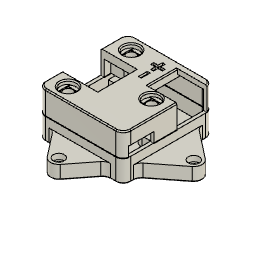
USB Adapter Mount (Autodesk Fusion 360 design; units mm, degrees)
Autodesk Fusion 360 part; units mm, degrees
note: some values were not read from the file. Chosen so that the rebuilt part matches the saved one: which face or edge a step refers to; which pieces of a blend or face edit are solid.
(part 1 of 2)
sketch "Sketch1" plane through (0, 0, 0) normal (0, 0, 1) x (1, 0, 0) in component "PCB"
  line L0 (0, 0) -> (27.432, 0)
  line L1 (27.432, 0) -> (27.432, 29.845)
  line L2 (27.432, 29.845) -> (0, 29.845)
  line L3 (0, 29.845) -> (0, 0)
  circle A0 centre (4.5, 3.5473) radius 1.6
  circle A1 centre (4.5, 26.5343) radius 1.6
  circle A2 centre (23.596, 14.865) radius 1.6
  line L4 (4.5, 26.5343) -> (4.5, 3.5473) construction
  dimension "d1" = 29.845
  dimension "d2" = 27.432
  dimension "d3" = 3.2
  dimension "d4" = 3.836
  dimension "d5" = 14.865
  dimension "d6" = 4.5
  dimension "d7" = 3.3107
  dimension "d8" = 3.5473
  constraint horizontal L0
  constraint vertical L1
  constraint horizontal L2
  constraint vertical L3
  constraint coincident L0.start L3.end
  constraint equal A0 A2
  constraint equal A0 A1
  constraint coincident A1.centre L4.start
  constraint vertical L4
  constraint coincident A0.centre L4.end
  measures "d1" distance of L0.end L1.end
  measures "d2" distance of L1.end L2.end
  measures "d3" diameter of A1
  measures "d4" distance of L1 A2.centre
  measures "d5" distance of L0 A2.centre
  measures "d6" distance of L3 L4
  measures "d7" distance of L2 A1.centre
  measures "d8" distance of L0 A0.centre
extrude "Extrude1" add sketch "Sketch1" along normal blind 1.6 makes body 1 in component "PCB"
fillet "Fillet1" radius 1.27 4 edges at (27.432, 0, 0.8) (0, 0, 0.8) (0, 29.845, 0.8) (27.432, 29.845, 0.8) on bodies 1 in component "PCB"
sketch "Sketch1 (2)" plane through (0, 0, 0) normal (0, 0, -1) x (1, 0, 0) in component "Mount"
  circle A0 centre (4.5, -26.5343) radius 1.6 construction
  circle A1 centre (4.5, -3.5473) radius 1.6 construction
  circle A2 centre (23.596, -14.865) radius 1.6 construction
  arc A3 (26.162, -29.845) -> (27.432, -28.575) centre (26.162, -28.575) ccw
  line L0 (27.432, -28.575) -> (27.432, -1.27) construction
  arc A4 (27.432, -1.27) -> (26.162, 0) centre (26.162, -1.27) ccw
  line L1 (26.162, 0) -> (1.27, 0) construction
  arc A5 (1.27, 0) -> (0, -1.27) centre (1.27, -1.27) ccw
  line L2 (0, -1.27) -> (0, -28.575) construction
  arc A6 (0, -28.575) -> (1.27, -29.845) centre (1.27, -28.575) ccw
  line L3 (1.27, -29.845) -> (26.162, -29.845) construction
  circle A7 centre (13.716, 9.0775) radius 1.2
  circle A8 centre (13.716, -22.4225) radius 1.2
  line L4 (13.716, 9.0775) -> (13.716, -22.4225) construction
  line L5 (0, -14.9225) -> (27.432, -14.9225) construction
  circle A9 centre (4.5, -3.5473) radius 1.4
  circle A10 centre (4.5, -26.5343) radius 1.4
  circle A11 centre (23.596, -14.865) radius 1.4
  circle A12 centre (4.5, -26.5343) radius 3.5
  circle A13 centre (23.596, -14.865) radius 3.5
  circle A14 centre (4.5, -3.5473) radius 3.5
  line L6 (6.325, -29.5208) -> (25.421, -17.8515)
  circle A15 centre (13.716, -22.4225) radius 3
  circle A16 centre (13.716, 9.0775) radius 3
  line L7 (1, -26.5343) -> (1, -3.5473)
  line L8 (6.2845, -0.5364) -> (25.3805, -11.8541)
  line L9 (16.716, 9.0775) -> (16.716, -22.4225)
  line L10 (1.7405, -1.3943) -> (11.3508, 10.9229)
  point P0 (13.716, -14.9225)
  dimension "d13" = 31.5
  dimension "d14" = 2.4
  dimension "d15" = 7.5
  dimension "d16" = 2.8
  dimension "d17" = 7
  dimension "d18" = 6
  constraint coincident A7.centre L4.start
  constraint vertical L4
  constraint coincident A8.centre L4.end
  constraint equal A7 A8
  constraint midpoint L2 L5.start
  constraint midpoint L0 L5.end
  constraint coincident L4 P0
  constraint midpoint L5 P0
  constraint concentric A1 A9
  constraint concentric A0 A10
  constraint concentric A2 A11
  constraint equal A9 A11
  constraint equal A9 A10
  constraint concentric A10 A12
  constraint concentric A11 A13
  constraint concentric A9 A14
  constraint equal A13 A14
  constraint equal A12 A14
  constraint coincident A12 L6.start
  constraint coincident A13 L6.end
  constraint tangent A13 L6
  constraint tangent A12 L6
  constraint concentric A8 A15
  constraint concentric A7 A16
  constraint equal A15 A16
  constraint coincident A12 L7.start
  constraint coincident A14 L7.end
  constraint perpendicular L5 L7
  constraint coincident A14 L8.start
  constraint coincident A13 L8.end
  constraint coincident A16 L9.start
  constraint coincident A15 L9.end
  constraint perpendicular L5 L9
  constraint tangent A16 L9
  constraint tangent A14 L8
  constraint tangent A13 L8
  constraint tangent A14 L7
  constraint coincident A14 L10.start
  constraint coincident A16 L10.end
  constraint tangent A16 L10
  constraint tangent A14 L10
  measures "d13" distance of A7.centre A8.centre
  measures "d14" diameter of A7
  measures "d15" distance of A8.centre P0
  measures "d16" diameter of A11
  measures "d17" diameter of A13
  measures "d18" diameter of A15
  measures "d37" angle of A2.centre
  measures "d99" angle of A2.centre
extrude "Extrude1'" add sketch "Sketch1 (2)" along normal blind 3 from surface at 3 separate body makes body 2 in component "Mount"
sketch "Sketch2" plane through (0, 0, -3) normal (0, 0, 1) x (-1, 0, 0) in component "Mount"
  circle A0 centre (-4.5, -3.5473) radius 1.4
  circle A1 centre (-23.596, -14.865) radius 1.4
  circle A2 centre (-13.716, -22.4225) radius 1.2
  circle A3 centre (-4.5, -26.5343) radius 1.4
  circle A4 centre (-13.716, 9.0775) radius 1.2
  arc A5 (-6.325, -29.5208) -> (-1, -26.5343) centre (-4.5, -26.5343) ccw
  line L0 (-1, -26.5343) -> (-1, -3.5473)
  arc A6 (-1, -3.5473) -> (-1.7405, -1.3943) centre (-4.5, -3.5473) ccw
  line L1 (-1.7405, -1.3943) -> (-11.3508, 10.9229)
  arc A7 (-11.3508, 10.9229) -> (-16.716, 9.0775) centre (-13.716, 9.0775) ccw
  line L2 (-16.716, 9.0775) -> (-16.716, -6.7189)
  line L3 (-16.716, -6.7189) -> (-25.3805, -11.8541)
  arc A8 (-25.3805, -11.8541) -> (-25.421, -17.8515) centre (-23.596, -14.865) ccw
  line L4 (-25.421, -17.8515) -> (-16.6023, -23.2405)
  arc A9 (-16.6023, -23.2405) -> (-13.1271, -25.3641) centre (-13.716, -22.4225) ccw
  line L5 (-13.1271, -25.3641) -> (-6.325, -29.5208)
  circle A10 centre (-13.716, -22.4225) radius 3
  circle A11 centre (-13.716, 9.0775) radius 3
  circle A12 centre (-13.716, 9.0775) radius 2
  circle A13 centre (-13.716, -22.4225) radius 2
  dimension "d22" = 4
  constraint concentric A2 A10
  constraint concentric A4 A11
  constraint concentric A11 A12
  constraint concentric A10 A13
  constraint equal A12 A13
  constraint tangent A9 A10
  constraint tangent A7 A11
  measures "d22" diameter of A13
extrude "Extrude2" add sketch "Sketch2" along normal blind 2 contours A9 A10 | A7 A11 bodies 2 in component "Mount"
sketch "Sketch3" plane through (0, 0, -3) normal (0, 0, 1) x (-1, 0, 0) in component "Mount"
  circle A0 centre (-4.5, -3.5473) radius 1.4
  circle A1 centre (-23.596, -14.865) radius 1.4
  circle A2 centre (-4.5, -26.5343) radius 1.4
  arc A3 (-13.1271, -25.3641) -> (-16.6023, -23.2405) centre (-13.716, -22.4225) ccw
  line L0 (-13.1271, -25.3641) -> (-6.325, -29.5208)
  arc A4 (-6.325, -29.5208) -> (-1, -26.5343) centre (-4.5, -26.5343) ccw
  line L1 (-1, -26.5343) -> (-1, -3.5473)
  arc A5 (-1, -3.5473) -> (-1.7405, -1.3943) centre (-4.5, -3.5473) ccw
  line L2 (-1.7405, -1.3943) -> (-11.3508, 10.9229)
  arc A6 (-16.716, 9.0775) -> (-11.3508, 10.9229) centre (-13.716, 9.0775) ccw
  line L3 (-16.716, 9.0775) -> (-16.716, -6.7189)
  line L4 (-16.716, -6.7189) -> (-25.3805, -11.8541)
  arc A7 (-25.3805, -11.8541) -> (-25.421, -17.8515) centre (-23.596, -14.865) ccw
  line L5 (-25.421, -17.8515) -> (-16.6023, -23.2405)
  circle A8 centre (-4.5, -3.5473) radius 3.5
  circle A9 centre (-23.596, -14.865) radius 3.5
  circle A10 centre (-4.5, -26.5343) radius 3.5
  constraint concentric A0 A8
  constraint concentric A1 A9
  constraint concentric A2 A10
  constraint tangent L0 A10
  constraint tangent L5 A9
  constraint tangent A5 A8
extrude "Extrude3" add sketch "Sketch3" along normal up to surface (3 mm away) contours A4 A10 | A7 A9 | A5 A8 bodies 2 in component "Mount"
sketch "Sketch1 (3)" plane through (0, 0, -3) normal (0, 0, 1) x (-1, 0, 0)
  arc A0 (-1, -26.5343) -> (-6.325, -29.5208) centre (-4.5, -26.5343) ccw
  line L0 (-1, -26.5343) -> (-1, -3.5473)
  arc A1 (-1.7405, -1.3943) -> (-1, -3.5473) centre (-4.5, -3.5473) ccw
  line L1 (-1.7405, -1.3943) -> (-11.3508, 10.9229)
  arc A2 (-16.716, 9.0775) -> (-11.3508, 10.9229) centre (-13.716, 9.0775) ccw
  line L2 (-16.716, 9.0775) -> (-16.716, -6.7189)
  line L3 (-16.716, -6.7189) -> (-25.3805, -11.8541)
  arc A3 (-25.421, -17.8515) -> (-25.3805, -11.8541) centre (-23.596, -14.865) ccw
  line L4 (-25.421, -17.8515) -> (-16.6023, -23.2405)
  arc A4 (-13.1271, -25.3641) -> (-16.6023, -23.2405) centre (-13.716, -22.4225) ccw
  line L5 (-13.1271, -25.3641) -> (-6.325, -29.5208)
  line L6 (1.5, -31.3343) -> (-29.596, -31.3343)
  line L7 (-29.596, -31.3343) -> (-29.596, 1.4527)
  line L8 (-29.596, 1.4527) -> (1.5, 1.4527)
  line L9 (1.5, 1.4527) -> (1.5, -31.3343)
  circle A5 centre (-4.5, -3.5473) radius 1.4
  circle A6 centre (-4.5, -26.5343) radius 1.4
  circle A7 centre (-23.596, -14.865) radius 1.4
  circle A8 centre (-13.716, -22.4225) radius 1.2
  arc A9 (-11.3508, 10.9229) -> (-16.716, 9.0775) centre (-13.716, 9.0775) ccw
  line L10 (-16.08, 10.9245) -> (-23.4802, 1.4527)
  dimension "d30" = 6
  dimension "d31" = 4.8
  dimension "d32" = 5
  dimension "d33" = 6
  dimension "d37" = 128
  constraint horizontal L6
  constraint vertical L7
  constraint horizontal L8
  constraint vertical L9
  constraint coincident A9 L10.start
  constraint coincident L8 L10.end
  constraint tangent A9 L10
  measures "d30" distance of A0.centre L9
  measures "d31" distance of A0.centre L6
  measures "d32" distance of A1.centre L8
  measures "d33" distance of A3.centre L7
  measures "d37" angle of L8 L10
extrude "Extrude4" add sketch "Sketch1 (3)" against normal up to surface (3 mm away) contours A0 L0 A1 L1 L2 L3 A3 L4 A4 L5 L6 L7 L8 L9 | L2 L8 A9 L10 bodies 2 in component "Mount"
sketch "Sketch4" plane through (0, 0, -3) normal (0, 0, 1) x (-1, 0, 0) in component "Mount"
  circle A0 centre (-23.596, -14.865) radius 3.5
  circle A1 centre (-13.716, -22.4225) radius 3
  circle A2 centre (-4.5, -26.5343) radius 3.5
  circle A3 centre (-4.5, -3.5473) radius 3.5
  arc A4 (-16.08, 10.9245) -> (-11.3508, 10.9229) centre (-13.716, 9.0775) ccw
  line L0 (-16.08, 10.9245) -> (-23.4802, 1.4527)
  line L1 (-23.4802, 1.4527) -> (-29.596, 1.4527)
  line L2 (-29.596, 1.4527) -> (-29.596, -31.3343)
  line L3 (-29.596, -31.3343) -> (1.5, -31.3343)
  line L4 (1.5, -31.3343) -> (1.5, 1.4527)
  line L5 (1.5, 1.4527) -> (-3.9618, 1.4527)
  line L6 (-3.9618, 1.4527) -> (-11.3508, 10.9229)
  line L7 (-23.596, -14.865) -> (-7.5, -14.865) construction
  line L8 (-23.596, -14.865) -> (-39, -14.865) construction
  circle A5 centre (-7.5, -14.865) radius 1.2
  circle A6 centre (-39, -14.865) radius 1.2
  circle A7 centre (-13.716, -22.4225) radius 1.2
  circle A8 centre (-39, -14.865) radius 3
  line L9 (-40.847, -17.229) -> (-29.596, -26.0193)
  line L10 (-40.847, -12.501) -> (-29.596, -3.7107)
  dimension "d94" = 31.5
  dimension "d95" = 31.5
  dimension "d96" = 8.9118
  dimension "d97" = 9
  dimension "d98" = 6
  dimension "d99" = 128
  constraint coincident A0.centre L7.start
  constraint horizontal L7
  constraint perpendicular L2 L8
  constraint coincident L7.end A5.centre
  constraint coincident L8.end A6.centre
  constraint equal A5 A6
  constraint equal A5 A7
  constraint concentric A6 A8
  constraint coincident A8 L9.start
  constraint coincident L2 L9.end
  constraint coincident A8 L10.start
  constraint coincident L2 L10.end
  constraint tangent A8 L10
  constraint tangent A8 L9
  constraint symmetric L8 L9 L10
  measures "d94" distance of A1.centre A4.centre
  measures "d95" distance of L7.end L8.end
  measures "d96" distance of L3 A1.centre
  measures "d97" distance of L4 L7.end
  measures "d98" diameter of A8
  measures "d99" angle of L2 L10
extrude "Extrude10" add sketch "Sketch4" against normal up to surface (3 mm away) contours L2 A8 L9 L10 | A8 bodies 2 in component "Mount"
extrude "Extrude11" cut sketch "Sketch4" against normal through all contours A5 bodies 2 in component "Mount"
sketch "Sketch6" plane through (0, 0, -3) normal (0, 0, 1) x (-1, 0, 0) in component "Mount"
  circle A0 centre (-7.5, -14.865) radius 1.2
  circle A1 centre (-39, -14.865) radius 1.2
  circle A2 centre (-23.596, -14.865) radius 3.5
  circle A3 centre (-13.716, -22.4225) radius 3
  circle A4 centre (-4.5, -26.5343) radius 3.5
  circle A5 centre (-4.5, -3.5473) radius 3.5
  arc A6 (-16.08, 10.9245) -> (-11.3508, 10.9229) centre (-13.716, 9.0775) ccw
  line L0 (-16.08, 10.9245) -> (-23.4802, 1.4527)
  line L1 (-23.4802, 1.4527) -> (-29.596, 1.4527)
  line L2 (-29.596, 1.4527) -> (-29.596, -3.7107)
  line L3 (-29.596, -3.7107) -> (-40.847, -12.501)
  arc A7 (-40.847, -12.501) -> (-40.847, -17.229) centre (-39, -14.865) ccw
  line L4 (-40.847, -17.229) -> (-29.596, -26.0193)
  line L5 (-29.596, -26.0193) -> (-29.596, -31.3343)
  line L6 (-29.596, -31.3343) -> (1.5, -31.3343)
  line L7 (1.5, -31.3343) -> (1.5, 1.4527)
  line L8 (1.5, 1.4527) -> (-3.9618, 1.4527)
  line L9 (-3.9618, 1.4527) -> (-11.3508, 10.9229)
  circle A8 centre (-7.5, -14.865) radius 3
  circle A9 centre (-7.5, -14.865) radius 2
  circle A10 centre (-39, -14.865) radius 3
  circle A11 centre (-39, -14.865) radius 2
  dimension "d104" = 4
  constraint concentric A0 A8
  constraint concentric A0 A9
  constraint equal A3 A8
  constraint concentric A1 A10
  constraint concentric A1 A11
  constraint equal A9 A11
  constraint equal A7 A10
  measures "d104" diameter of A9
extrude "Extrude12" add sketch "Sketch6" along normal up to surface (2 mm away) contours A7 A10 | A8 bodies 2 in component "Mount"
fillet "Fillet2" radius 2.77 4 edges at (-1.5, -1.4527, -4.5) (29.596, -1.4527, -4.5) (29.596, 31.3343, -4.5) (-1.5, 31.3343, -4.5) on bodies 2 in component "Mount"
sketch "Sketch2 (2)" plane through (0, 0, -3) normal (0, 0, 1) x (-1, 0, 0)
  line L0 (-3.9618, 1.4527) -> (-23.4802, 1.4527)
  line L1 (0.3, -28.5643) -> (0.3, -1.3173)
  arc A0 (0.3, -1.3173) -> (-1.27, 0.2527) centre (-1.27, -1.3173) ccw
  line L2 (-1.27, 0.2527) -> (-4.5476, 0.2527)
  arc A1 (-17.4707, 7.1954) -> (-9.9626, 7.1929) centre (-13.716, 9.0775) ccw
  line L3 (-22.8949, 0.2527) -> (-26.826, 0.2527)
  arc A2 (-26.826, 0.2527) -> (-28.396, -1.3173) centre (-26.826, -1.3173) ccw
  line L4 (-28.396, -1.3173) -> (-28.396, -28.5643)
  arc A3 (-28.396, -28.5643) -> (-26.826, -30.1343) centre (-26.826, -28.5643) ccw
  line L5 (-26.826, -30.1343) -> (-1.27, -30.1343)
  arc A4 (-1.27, -30.1343) -> (0.3, -28.5643) centre (-1.27, -28.5643) ccw
  line L6 (-4.5476, 0.2527) -> (-22.8949, 0.2527)
  circle A5 centre (-13.716, -22.4225) radius 2
  circle A6 centre (-13.716, -22.4225) radius 1.2
  constraint tangent L1 A4
  constraint tangent L3 A2
  constraint tangent L1 A0
  constraint tangent A0 L2
  constraint tangent A2 L4
  constraint tangent L4 A3
  constraint tangent A3 L5
  constraint tangent L5 A4
  constraint parallel L3 L6
sketch "Sketch7" plane through (0, 0, -3) normal (0, 0, 1) x (-1, 0, 0) in component "Mount"
  arc A0 (-1.27, -31.3343) -> (1.5, -28.5643) centre (-1.27, -28.5643) ccw
  line L0 (1.5, -28.5643) -> (1.5, -1.3173)
  arc A1 (1.5, -1.3173) -> (-1.27, 1.4527) centre (-1.27, -1.3173) ccw
  line L1 (-1.27, 1.4527) -> (-3.9618, 1.4527)
  line L2 (-3.9618, 1.4527) -> (-11.3508, 10.9229)
  arc A2 (-16.08, 10.9245) -> (-11.3508, 10.9229) centre (-13.716, 9.0775) ccw
  line L3 (-16.08, 10.9245) -> (-23.4802, 1.4527)
  line L4 (-23.4802, 1.4527) -> (-26.826, 1.4527)
  arc A3 (-26.826, 1.4527) -> (-29.596, -1.3173) centre (-26.826, -1.3173) ccw
  line L5 (-29.596, -1.3173) -> (-29.596, -3.7107)
  line L6 (-29.596, -3.7107) -> (-40.847, -12.501)
  arc A4 (-40.847, -17.229) -> (-40.847, -12.501) centre (-39, -14.865) ccw
  line L7 (-40.847, -17.229) -> (-29.596, -26.0193)
  line L8 (-29.596, -26.0193) -> (-29.596, -28.5643)
  arc A5 (-29.596, -28.5643) -> (-26.826, -31.3343) centre (-26.826, -28.5643) ccw
  line L9 (-26.826, -31.3343) -> (-1.27, -31.3343)
  circle A6 centre (-4.5, -3.5473) radius 3.5
  circle A7 centre (-4.5, -26.5343) radius 3.5
  circle A8 centre (-13.716, -22.4225) radius 3
  circle A9 centre (-23.596, -14.865) radius 3.5
  circle A10 centre (-7.5, -14.865) radius 3
  line L10 (-3.9618, 1.4527) -> (-23.4802, 1.4527)
  line L11 (-29.596, -3.7107) -> (-29.596, -26.0193)
  line L12 (0.3, -28.5643) -> (0.3, -1.3173)
  arc A11 (0.3, -1.3173) -> (-1.27, 0.2527) centre (-1.27, -1.3173) ccw
  line L13 (-1.27, 0.2527) -> (-4.5476, 0.2527)
  line L14 (-4.5476, 0.2527) -> (-9.9626, 7.1929)
  arc A12 (-17.4707, 7.1954) -> (-9.9626, 7.1929) centre (-13.716, 9.0775) ccw
  line L15 (-17.4707, 7.1954) -> (-22.8949, 0.2527)
  line L16 (-22.8949, 0.2527) -> (-26.826, 0.2527)
  arc A13 (-26.826, 0.2527) -> (-28.396, -1.3173) centre (-26.826, -1.3173) ccw
  line L17 (-28.396, -1.3173) -> (-28.396, -4.296)
  line L18 (-28.396, -4.296) -> (-37.1179, -11.1103)
  arc A14 (-37.1179, -18.6197) -> (-37.1179, -11.1103) centre (-39, -14.865) ccw
  line L19 (-37.1179, -18.6197) -> (-28.396, -25.434)
  line L20 (-28.396, -25.434) -> (-28.396, -28.5643)
  arc A15 (-28.396, -28.5643) -> (-26.826, -30.1343) centre (-26.826, -28.5643) ccw
  line L21 (-26.826, -30.1343) -> (-1.27, -30.1343)
  arc A16 (-1.27, -30.1343) -> (0.3, -28.5643) centre (-1.27, -28.5643) ccw
  line L22 (-28.396, -25.434) -> (-28.396, -4.296)
  line L23 (-22.8949, 0.2527) -> (-4.5476, 0.2527)
  dimension "d107" = -1.2
  constraint coincident L1.end L2.start
  constraint coincident L3.end L4.start
  constraint coincident L5.end L6.start
  constraint coincident L7.end L8.start
extrude "Extrude5" add sketch "Sketch7" along normal up to surface (5.2 mm away) contours A0 L0 A1 L1 L8 A5 L9 L10 L11 L12 A11 L13 L14 L19 L20 A15 L21 A16 | L11 L18 L19 L22 | L10 L14 L15 L23 | L4 A3 L5 L10 L11 L15 L16 A13 L17 L18 bodies 2 in component "Mount"
sketch "Sketch3 (2)" plane through (0, 0, 0) normal (0, 0, 1) x (-1, 0, 0)
  circle A0 centre (-23.596, -14.865) radius 1.4
  circle A1 centre (-23.596, -14.865) radius 3.5
  circle A2 centre (-4.5, -3.5473) radius 3.5
  circle A3 centre (-4.5, -26.5343) radius 3.5
  line L0 (-23.596, -18.365) -> (-28.396, -18.365)
  line L1 (-23.596, -11.365) -> (-28.396, -11.365)
  line L2 (-8, -3.5473) -> (-8, 0.2527)
  line L3 (-4.5, -7.0473) -> (0.3, -7.0473)
  line L4 (-4.5, -23.0343) -> (0.3, -23.0343)
  line L5 (-8, -26.5343) -> (-8, -30.1343)
  line L6 (-28.396, -1.3173) -> (-28.396, -28.5643)
  line L7 (0.3, -28.5643) -> (0.3, -1.3173)
  line L8 (-1.27, 0.2527) -> (-26.826, 0.2527)
  line L9 (-26.826, -30.1343) -> (-1.27, -30.1343)
  arc A4 (0.3, -1.3173) -> (-1.27, 0.2527) centre (-1.27, -1.3173) ccw
  arc A5 (-26.826, 0.2527) -> (-28.396, -1.3173) centre (-26.826, -1.3173) ccw
  arc A6 (-28.396, -28.5643) -> (-26.826, -30.1343) centre (-26.826, -28.5643) ccw
  arc A7 (-1.27, -30.1343) -> (0.3, -28.5643) centre (-1.27, -28.5643) ccw
  constraint coincident A1 L0.start
  constraint coincident L0.end L6
  constraint perpendicular L0 L6
  constraint coincident A1 L1.start
  constraint coincident L1.end L6
  constraint perpendicular L1 L6
  constraint coincident A2 L2.start
  constraint coincident L2.end L8
  constraint perpendicular L2 L8
  constraint coincident A2 L3.start
  constraint coincident L3.end L7
  constraint perpendicular L3 L7
  constraint coincident A3 L4.start
  constraint coincident L4.end L7
  constraint perpendicular L4 L7
  constraint coincident A3 L5.start
  constraint coincident L5.end L9
  constraint perpendicular L5 L9
  constraint tangent A2 L3
  constraint tangent A2 L2
  constraint tangent A1 L1
  constraint tangent A1 L0
  constraint tangent A3 L5
  constraint tangent A3 L4
sketch "Sketch8" plane through (0, 0, -3) normal (0, 0, 1) x (-1, 0, 0) in component "Mount"
  line L0 (0.3, -28.5643) -> (0.3, -1.3173)
  arc A0 (0.3, -1.3173) -> (-1.27, 0.2527) centre (-1.27, -1.3173) ccw
  line L1 (-1.27, 0.2527) -> (-26.826, 0.2527)
  arc A1 (-26.826, 0.2527) -> (-28.396, -1.3173) centre (-26.826, -1.3173) ccw
  line L2 (-28.396, -1.3173) -> (-28.396, -28.5643)
  arc A2 (-28.396, -28.5643) -> (-26.826, -30.1343) centre (-26.826, -28.5643) ccw
  line L3 (-26.826, -30.1343) -> (-1.27, -30.1343)
  arc A3 (-1.27, -30.1343) -> (0.3, -28.5643) centre (-1.27, -28.5643) ccw
  circle A4 centre (-4.5, -3.5473) radius 3.5
  circle A5 centre (-4.5, -26.5343) radius 3.5
  circle A6 centre (-13.716, -22.4225) radius 3
  circle A7 centre (-23.596, -14.865) radius 3.5
  circle A8 centre (-7.5, -14.865) radius 3
  line L4 (-4.5, -23.0343) -> (0.3, -23.0343)
  line L5 (-8, -26.5343) -> (-8, -30.1343)
  line L6 (-8, -3.5473) -> (-8, 0.2527)
  line L7 (-4.5, -7.0473) -> (0.3, -7.0473)
  line L8 (-23.596, -11.365) -> (-28.396, -11.365)
  line L9 (-23.596, -18.365) -> (-28.396, -18.365)
  constraint coincident A5 L4.start
  constraint coincident L0 L4.end
  constraint perpendicular L0 L4
  constraint coincident A5 L5.start
  constraint coincident L3 L5.end
  constraint perpendicular L3 L5
  constraint coincident A4 L6.start
  constraint coincident L1 L6.end
  constraint perpendicular L1 L6
  constraint coincident L0 L7.end
  constraint perpendicular L0 L7
  constraint coincident A7 L8.start
  constraint coincident L2 L8.end
  constraint perpendicular L2 L8
  constraint coincident A7 L9.start
  constraint coincident L2 L9.end
  constraint perpendicular L2 L9
  constraint tangent A5 L4
  constraint tangent A5 L5
  constraint tangent A4 L6
  constraint tangent A4 L7
  constraint tangent A7 L8
  constraint tangent A7 L9
  constraint coincident A4 L7.start
extrude "Extrude6" add sketch "Sketch3 (2)" against normal up to surface (3 mm away) contours A1 L0 L1 L6 | A2 L2 L3 L7 L8 A4 | A3 L4 L5 L7 L9 A7 bodies 2 in component "Mount"
extrude "Extrude8" add 6 faces at (0.139, 4.085, 0) (0.139, 25.9299, 0) (27.9594, 14.7778, 0) (25.6438, 12.965, 0) (4.2939, 23.7482, 0) (4.2939, 6.3334, 0) along direction (0, 0, 1) blind 0.6 on bodies 2 bodies 2 in component "Mount"
extrude "Extrude7" add 2 faces at (13.7583, -2.9951, -3) (31.7307, 14.865, -3) along direction (0, 0, 1) up to surface end surface through (0, 0, -1) normal (0, 0, 1) offset 0 on bodies 2 bodies 2 in component "Mount"
fillet "Fillet3" radius 1 4 edges at (15.2803, 24.9824, -3) (11.3958, 24.3243, -3) (14.1289, 19.4511, -3) (10.5, 14.865, -3) on bodies 2 in component "Mount"
fillet "Fillet4" radius 3 4 edges at (3.9618, -1.4527, -3.5) (23.4802, -1.4527, -3.5) (29.596, 3.7107, -3.5) (29.596, 26.0193, -3.5) on bodies 2 in component "Mount"
chamfer "Chamfer2" distance 0.4 angle 45 1 faces at (17.1485, 5.0703, -6) on bodies 2 in component "Mount"
sketch "Sketch1 (4)" plane through (0, 0, 2.2) normal (0, 0, 1) x (-1, 0, 0) in component "Cover"
  arc A0 (1.5, -1.3173) -> (-1.27, 1.4527) centre (-1.27, -1.3173) ccw
  line L0 (-1.27, 1.4527) -> (-26.826, 1.4527)
  arc A1 (-26.826, 1.4527) -> (-29.596, -1.3173) centre (-26.826, -1.3173) ccw
  line L1 (-29.596, -1.3173) -> (-29.596, -28.5643)
  arc A2 (-29.596, -28.5643) -> (-26.826, -31.3343) centre (-26.826, -28.5643) ccw
  line L2 (-26.826, -31.3343) -> (-1.27, -31.3343)
  arc A3 (-1.27, -31.3343) -> (1.5, -28.5643) centre (-1.27, -28.5643) ccw
  line L3 (1.5, -28.5643) -> (1.5, -1.3173)
  line L4 (-28.396, -28.5643) -> (-28.396, -1.3173)
  arc A4 (-26.826, 0.2527) -> (-28.396, -1.3173) centre (-26.826, -1.3173) ccw
  line L5 (-26.826, 0.2527) -> (-1.27, 0.2527)
  arc A5 (0.3, -1.3173) -> (-1.27, 0.2527) centre (-1.27, -1.3173) ccw
  line L6 (0.3, -1.3173) -> (0.3, -28.5643)
  arc A6 (-1.27, -30.1343) -> (0.3, -28.5643) centre (-1.27, -28.5643) ccw
  line L7 (-1.27, -30.1343) -> (-26.826, -30.1343)
  arc A7 (-28.396, -28.5643) -> (-26.826, -30.1343) centre (-26.826, -28.5643) ccw
extrude "Extrude1''" add sketch "Sketch1 (4)" along normal blind 6.8 separate body contours A0 L0 A1 L1 A2 L2 A3 L3 | L4 A4 L5 A5 L6 A6 L7 A7 makes body 3 in component "Cover"
shell "Shell1" thickness 1.2 removed faces 1 at (19.2307, 10.3996, 2.2) on bodies 3 in component "Cover"
sketch "Sketch2 (3)" plane through (0, 0, 9) normal (0, 0, 1) x (-1, 0, 0) in component "Cover"
  line L0 (1.5, -28.5643) -> (1.5, -1.3173)
  arc A0 (1.5, -1.3173) -> (-1.27, 1.4527) centre (-1.27, -1.3173) ccw
  line L1 (-1.27, 1.4527) -> (-26.826, 1.4527)
  arc A1 (-26.826, 1.4527) -> (-29.596, -1.3173) centre (-26.826, -1.3173) ccw
  line L2 (-29.596, -1.3173) -> (-29.596, -28.5643)
  arc A2 (-29.596, -28.5643) -> (-26.826, -31.3343) centre (-26.826, -28.5643) ccw
  line L3 (-26.826, -31.3343) -> (-1.27, -31.3343)
  arc A3 (-1.27, -31.3343) -> (1.5, -28.5643) centre (-1.27, -28.5643) ccw
  circle A4 centre (-4.5, -26.5343) radius 1.4 construction
  circle A5 centre (-23.596, -14.865) radius 1.4 construction
  circle A6 centre (-4.5, -3.5473) radius 1.4 construction
  circle A7 centre (-23.596, -14.865) radius 1.65
  circle A8 centre (-4.5, -3.5473) radius 1.65
  circle A9 centre (-4.5, -26.5343) radius 1.65
  dimension "d83" = 3.3
  constraint concentric A5 A7
  constraint concentric A6 A8
  constraint concentric A4 A9
  constraint equal A8 A9
  constraint equal A7 A8
  measures "d83" diameter of A7
extrude "Extrude2'" cut sketch "Sketch2 (3)" against normal up to surface (1.2 mm away) contours A7 | A8 | A9 bodies 3 in component "Cover"
sketch "Sketch3 (3)" plane through (0, 0, 7.8) normal (0, 0, -1) x (1, 0, 0) in component "Cover"
  line L0 (-0.3, -1.3173) -> (-0.3, -28.5643)
  arc A0 (-0.3, -28.5643) -> (1.27, -30.1343) centre (1.27, -28.5643) ccw
  line L1 (1.27, -30.1343) -> (26.826, -30.1343)
  arc A1 (26.826, -30.1343) -> (28.396, -28.5643) centre (26.826, -28.5643) ccw
  line L2 (28.396, -28.5643) -> (28.396, -1.3173)
  arc A2 (28.396, -1.3173) -> (26.826, 0.2527) centre (26.826, -1.3173) ccw
  line L3 (26.826, 0.2527) -> (1.27, 0.2527)
  arc A3 (1.27, 0.2527) -> (-0.3, -1.3173) centre (1.27, -1.3173) ccw
  circle A4 centre (4.5, -3.5473) radius 2.6
  circle A5 centre (4.5, -26.5343) radius 2.6
  circle A6 centre (23.596, -14.865) radius 2.6
  line L4 (4.5, -6.1473) -> (-0.3, -6.1473)
  line L5 (7.1, -3.5473) -> (7.1, 0.2527)
  line L6 (4.5, -23.9343) -> (-0.3, -23.9343)
  line L7 (7.1, -26.5343) -> (7.1, -30.1343)
  line L8 (23.596, -17.465) -> (28.396, -17.465)
  line L9 (23.596, -12.265) -> (28.396, -12.265)
  circle A7 centre (23.596, -14.865) radius 1.65
  circle A8 centre (4.5, -26.5343) radius 1.65
  circle A9 centre (4.5, -3.5473) radius 1.65
  dimension "d59" = 5.2
  constraint equal A4 A6
  constraint equal A5 A6
  constraint coincident A4 L4.start
  constraint coincident L0 L4.end
  constraint perpendicular L0 L4
  constraint coincident A4 L5.start
  constraint coincident L3 L5.end
  constraint perpendicular L3 L5
  constraint coincident A5 L6.start
  constraint coincident L0 L6.end
  constraint perpendicular L0 L6
  constraint coincident A5 L7.start
  constraint coincident L1 L7.end
  constraint perpendicular L1 L7
  constraint coincident A6 L8.start
  constraint coincident L2 L8.end
  constraint perpendicular L2 L8
  constraint coincident A6 L9.start
  constraint coincident L2 L9.end
  constraint perpendicular L2 L9
  constraint tangent A4 L4
  constraint tangent A4 L5
  constraint tangent A5 L6
  constraint tangent A5 L7
  constraint tangent A6 L9
  constraint tangent A6 L8
  constraint coincident A6.centre A7.centre
  constraint coincident A4.centre A9.centre
  constraint coincident A5.centre A8.centre
  measures "d59" diameter of A4
extrude "Extrude3'" add sketch "Sketch3 (3)" along normal up to surface (5.6 mm away) contours L0 L3 A3 A4 L4 L5 | L0 A0 L1 A5 L6 L7 | A4 | A5 | L2 A6 L8 L9 | A6 bodies 3 in component "Cover"
sketch "Sketch4 (2)" plane through (0, 0, 9) normal (0, 0, 1) x (-1, 0, 0) in component "Cover"
  line L0 (1.5, -28.5643) -> (1.5, -1.3173)
  arc A0 (1.5, -1.3173) -> (-1.27, 1.4527) centre (-1.27, -1.3173) ccw
  line L1 (-1.27, 1.4527) -> (-26.826, 1.4527)
  arc A1 (-26.826, 1.4527) -> (-29.596, -1.3173) centre (-26.826, -1.3173) ccw
  line L2 (-29.596, -1.3173) -> (-29.596, -28.5643)
  arc A2 (-29.596, -28.5643) -> (-26.826, -31.3343) centre (-26.826, -28.5643) ccw
  line L3 (-26.826, -31.3343) -> (-1.27, -31.3343)
  arc A3 (-1.27, -31.3343) -> (1.5, -28.5643) centre (-1.27, -28.5643) ccw
  circle A4 centre (-4.5, -26.5343) radius 2.9
  circle A5 centre (-4.5, -3.5473) radius 2.9
  circle A6 centre (-23.596, -14.865) radius 2.9
  circle A7 centre (-23.596, -14.865) radius 1.65
  circle A8 centre (-4.5, -26.5343) radius 1.65
  circle A9 centre (-4.5, -3.5473) radius 1.65
  dimension "d63" = 5.8
  constraint equal A4 A5
  constraint equal A4 A6
  constraint coincident A6.centre A7.centre
  constraint coincident A5.centre A9.centre
  constraint coincident A4.centre A8.centre
  measures "d63" diameter of A6
extrude "Extrude4'" add sketch "Sketch4 (2)" along normal blind 1.6 contours L0 A0 L1 A1 L2 A2 L3 A3 bodies 3 in component "Cover"
sketch "Sketch6 (2)" plane through (0, 0, 2.2) normal (0, 0, -1) x (1, 0, 0) in component "Cover"
  line L0 (-0.3, -23.9343) -> (-0.3, -6.1473)
  line L1 (-0.3, -6.1473) -> (4.5, -6.1473)
  arc A0 (4.5, -6.1473) -> (7.1, -3.5473) centre (4.5, -3.5473) ccw
  line L2 (7.1, -3.5473) -> (7.1, 0.2527)
  line L3 (7.1, 0.2527) -> (26.826, 0.2527)
  arc A1 (28.396, -1.3173) -> (26.826, 0.2527) centre (26.826, -1.3173) ccw
  line L4 (28.396, -1.3173) -> (28.396, -12.265)
  line L5 (28.396, -12.265) -> (23.596, -12.265)
  arc A2 (23.596, -12.265) -> (23.596, -17.465) centre (23.596, -14.865) ccw
  line L6 (23.596, -17.465) -> (28.396, -17.465)
  line L7 (28.396, -17.465) -> (28.396, -28.5643)
  arc A3 (26.826, -30.1343) -> (28.396, -28.5643) centre (26.826, -28.5643) ccw
  line L8 (26.826, -30.1343) -> (7.1, -30.1343)
  line L9 (7.1, -30.1343) -> (7.1, -26.5343)
  arc A4 (7.1, -26.5343) -> (4.5, -23.9343) centre (4.5, -26.5343) ccw
  line L10 (4.5, -23.9343) -> (-0.3, -23.9343)
  line L11 (-1.5, -1.3173) -> (-1.5, -28.5643)
  arc A5 (-1.5, -28.5643) -> (1.27, -31.3343) centre (1.27, -28.5643) ccw
  line L12 (1.27, -31.3343) -> (26.826, -31.3343)
  arc A6 (26.826, -31.3343) -> (29.596, -28.5643) centre (26.826, -28.5643) ccw
  line L13 (29.596, -28.5643) -> (29.596, -1.3173)
  arc A7 (29.596, -1.3173) -> (26.826, 1.4527) centre (26.826, -1.3173) ccw
  line L14 (26.826, 1.4527) -> (1.27, 1.4527)
  arc A8 (1.27, 1.4527) -> (-1.5, -1.3173) centre (1.27, -1.3173) ccw
  line L15 (-1.5, -7.1473) -> (-0.3, -7.1473)
  line L16 (-1.5, -21.5343) -> (-0.3, -21.5343)
  circle A9 centre (4.5, -3.5473) radius 1.65
  circle A10 centre (4.5, -26.5343) radius 1.65
  circle A11 centre (23.596, -14.865) radius 1.65
  dimension "d67" = 7.4
  dimension "d68" = 8.6
  dimension "d111" = 14.387
  constraint coincident L11 L15.start
  constraint coincident L0 L15.end
  constraint perpendicular L0 L15
  constraint coincident L11 L16.start
  constraint coincident L0 L16.end
  constraint perpendicular L0 L16
  measures "d67" distance of L3 L15.end
  measures "d68" distance of L8 L16.end
  measures "d111" distance of L15.start L16.start
extrude "Extrude5'" cut sketch "Sketch6 (2)" against normal up to surface (8.4 mm away) contours L0 L11 L15 L16 bodies 3 in component "Cover"
sketch "Sketch7 (2)" plane through (0, 0, 2.2) normal (0, 0, -1) x (1, 0, 0) in component "Cover"
  line L0 (-0.3, -21.5343) -> (-1.5, -21.5343)
  line L1 (-1.5, -21.5343) -> (-1.5, -28.5643)
  arc A0 (-1.5, -28.5643) -> (1.27, -31.3343) centre (1.27, -28.5643) ccw
  line L2 (1.27, -31.3343) -> (26.826, -31.3343)
  arc A1 (26.826, -31.3343) -> (29.596, -28.5643) centre (26.826, -28.5643) ccw
  line L3 (29.596, -28.5643) -> (29.596, -1.3173)
  arc A2 (29.596, -1.3173) -> (26.826, 1.4527) centre (26.826, -1.3173) ccw
  line L4 (26.826, 1.4527) -> (1.27, 1.4527)
  arc A3 (1.27, 1.4527) -> (-1.5, -1.3173) centre (1.27, -1.3173) ccw
  line L5 (-1.5, -1.3173) -> (-1.5, -7.1473)
  line L6 (-1.5, -7.1473) -> (-0.3, -7.1473)
  line L7 (-0.3, -7.1473) -> (-0.3, -6.1473)
  line L8 (-0.3, -6.1473) -> (4.5, -6.1473)
  arc A4 (4.5, -6.1473) -> (7.1, -3.5473) centre (4.5, -3.5473) ccw
  line L9 (7.1, -3.5473) -> (7.1, 0.2527)
  line L10 (7.1, 0.2527) -> (26.826, 0.2527)
  arc A5 (28.396, -1.3173) -> (26.826, 0.2527) centre (26.826, -1.3173) ccw
  line L11 (28.396, -1.3173) -> (28.396, -12.265)
  line L12 (28.396, -12.265) -> (23.596, -12.265)
  arc A6 (23.596, -12.265) -> (23.596, -17.465) centre (23.596, -14.865) ccw
  line L13 (23.596, -17.465) -> (28.396, -17.465)
  line L14 (28.396, -17.465) -> (28.396, -28.5643)
  arc A7 (26.826, -30.1343) -> (28.396, -28.5643) centre (26.826, -28.5643) ccw
  line L15 (26.826, -30.1343) -> (7.1, -30.1343)
  line L16 (7.1, -30.1343) -> (7.1, -26.5343)
  arc A8 (7.1, -26.5343) -> (4.5, -23.9343) centre (4.5, -26.5343) ccw
  line L17 (4.5, -23.9343) -> (-0.3, -23.9343)
  line L18 (-0.3, -23.9343) -> (-0.3, -21.5343)
  line L19 (28.396, -9.7473) -> (29.596, -9.7473)
  line L20 (28.1942, -0.5473) -> (29.4868, -0.5473)
  circle A9 centre (23.596, -14.865) radius 1.65
  circle A10 centre (4.5, -26.5343) radius 1.65
  circle A11 centre (4.5, -3.5473) radius 1.65
  dimension "d73" = 0.8
  dimension "d74" = 9.2
  constraint coincident L11 L19.start
  constraint coincident L3 L19.end
  constraint perpendicular L3 L19
  constraint coincident A5 L20.start
  constraint coincident A2 L20.end
  constraint horizontal L20
  measures "d73" distance of L10 L20.start
  measures "d74" vertical distance of L19.end L20.end
extrude "Extrude6'" cut sketch "Sketch7 (2)" against normal blind 3.6 contours L3 A2 A5 L11 L19 L20 bodies 3 in component "Cover"
sketch "Sketch8 (2)" plane through (0, 0, 2.2) normal (0, 0, -1) x (1, 0, 0) in component "Cover"
  line L0 (29.596, -9.7473) -> (28.396, -9.7473)
  line L1 (28.396, -9.7473) -> (28.396, -12.265)
  line L2 (28.396, -12.265) -> (23.596, -12.265)
  arc A0 (23.596, -12.265) -> (23.596, -17.465) centre (23.596, -14.865) ccw
  line L3 (23.596, -17.465) -> (28.396, -17.465)
  line L4 (28.396, -17.465) -> (28.396, -28.5643)
  arc A1 (26.826, -30.1343) -> (28.396, -28.5643) centre (26.826, -28.5643) ccw
  line L5 (26.826, -30.1343) -> (7.1, -30.1343)
  line L6 (7.1, -30.1343) -> (7.1, -26.5343)
  arc A2 (7.1, -26.5343) -> (4.5, -23.9343) centre (4.5, -26.5343) ccw
  line L7 (4.5, -23.9343) -> (-0.3, -23.9343)
  line L8 (-0.3, -23.9343) -> (-0.3, -21.5343)
  line L9 (-0.3, -21.5343) -> (-1.5, -21.5343)
  line L10 (-1.5, -21.5343) -> (-1.5, -28.5643)
  arc A3 (-1.5, -28.5643) -> (1.27, -31.3343) centre (1.27, -28.5643) ccw
  line L11 (1.27, -31.3343) -> (26.826, -31.3343)
  arc A4 (26.826, -31.3343) -> (29.596, -28.5643) centre (26.826, -28.5643) ccw
  line L12 (29.596, -28.5643) -> (29.596, -9.7473)
  line L13 (29.596, -18.1343) -> (18.796, -18.1343)
  line L14 (18.796, -18.1343) -> (18.796, -29.1343)
  line L15 (18.796, -29.1343) -> (33.5882, -29.1343)
  circle A5 centre (23.596, -14.865) radius 1.65
  circle A6 centre (4.5, -26.5343) radius 1.65
  dimension "d77" = 11
  dimension "d78" = 12
  dimension "d79" = 9.6
  constraint coincident L12 L13.start
  constraint perpendicular L4 L13
  constraint perpendicular L13 L14
  constraint perpendicular L14 L15
  measures "d77" distance of L13.end L14.end
  measures "d78" vertical distance of A1.start L13.start
  measures "d79" distance of L4 L14
extrude "Extrude7'" cut sketch "Sketch8 (2)" against normal through all contours L4 A1 A4 L12 L13 L15 | L4 A1 L13 L14 L15 bodies 3 in component "Cover"
sketch "Sketch14" plane through (0, 0, 10.6) normal (0, 0, 1) x (-1, 0, 0) in component "Cover"
  circle A0 centre (-4.5, -26.5343) radius 2.9
  circle A1 centre (-4.5, -3.5473) radius 2.9
  circle A2 centre (-23.596, -14.865) radius 2.9
  line L0 (-29.596, -18.1343) -> (-18.796, -18.1343)
  line L1 (-18.796, -18.1343) -> (-18.796, -29.1343)
  line L2 (-18.796, -29.1343) -> (-29.5367, -29.1343)
  arc A3 (-29.5367, -29.1343) -> (-26.826, -31.3343) centre (-26.826, -28.5643) ccw
  line L3 (-26.826, -31.3343) -> (-1.27, -31.3343)
  arc A4 (-1.27, -31.3343) -> (1.5, -28.5643) centre (-1.27, -28.5643) ccw
  line L4 (1.5, -28.5643) -> (1.5, -21.5343)
  line L5 (1.5, -21.5343) -> (0.3, -21.5343)
  line L6 (0.3, -21.5343) -> (0.3, -7.1473)
  line L7 (0.3, -7.1473) -> (1.5, -7.1473)
  line L8 (1.5, -7.1473) -> (1.5, -1.3173)
  arc A5 (1.5, -1.3173) -> (-1.27, 1.4527) centre (-1.27, -1.3173) ccw
  line L9 (-1.27, 1.4527) -> (-26.826, 1.4527)
  arc A6 (-26.826, 1.4527) -> (-29.596, -1.3173) centre (-26.826, -1.3173) ccw
  line L10 (-29.596, -1.3173) -> (-29.596, -18.1343)
  line L11 (-18.796, -23.6343) -> (-14.696, -23.6343) construction
  line L12 (-14.696, -23.6343) -> (-14.696, -26.1343) construction
  line L13 (-15.196, -24.0343) -> (-15.196, -25.6343)
  line L14 (-15.196, -25.6343) -> (-16.796, -25.6343)
  line L15 (-16.796, -25.6343) -> (-16.796, -26.6343)
  line L16 (-16.796, -26.6343) -> (-15.196, -26.6343)
  line L17 (-15.196, -26.6343) -> (-15.196, -28.2343)
  line L18 (-15.196, -28.2343) -> (-14.196, -28.2343)
  line L19 (-14.196, -28.2343) -> (-14.196, -26.6343)
  line L20 (-14.196, -26.6343) -> (-12.596, -26.6343)
  line L21 (-12.596, -26.6343) -> (-12.596, -25.6343)
  line L22 (-12.596, -25.6343) -> (-14.196, -25.6343)
  line L23 (-14.196, -25.6343) -> (-14.196, -24.0343)
  line L24 (-14.196, -24.0343) -> (-15.196, -24.0343)
  line L25 (-15.196, -25.6343) -> (-14.196, -26.6343) construction
  line L26 (-14.696, -23.6343) -> (-14.696, -21.1343) construction
  line L27 (-15.196, -19.5343) -> (-15.196, -22.7343)
  line L28 (-15.196, -22.7343) -> (-14.196, -22.7343)
  line L29 (-14.196, -22.7343) -> (-14.196, -19.5343)
  line L30 (-14.196, -19.5343) -> (-15.196, -19.5343)
  line L31 (-15.196, -21.1343) -> (-14.196, -21.1343) construction
  dimension "d119" = 2.5
  dimension "d120" = 1
  dimension "d121" = 1.6
  dimension "d123" = 2
  dimension "d127" = 3.2
  constraint midpoint L1 L11.start
  constraint perpendicular L1 L11
  constraint perpendicular L11 L12
  constraint perpendicular L11 L13
  constraint perpendicular L13 L14
  constraint perpendicular L14 L15
  constraint perpendicular L15 L16
  constraint perpendicular L16 L17
  constraint perpendicular L17 L18
  constraint perpendicular L18 L19
  constraint perpendicular L19 L20
  constraint perpendicular L20 L21
  constraint perpendicular L19 L22
  constraint perpendicular L11 L23
  constraint perpendicular L12 L24
  constraint coincident L13.start L24.end
  constraint collinear L14 L22
  constraint collinear L16 L20
  constraint collinear L19 L23
  constraint collinear L13 L17
  constraint equal L19 L20
  constraint equal L22 L23
  constraint equal L13 L14
  constraint equal L18 L21
  constraint coincident L12.end L25
  constraint midpoint L12.end L25
  constraint perpendicular L11 L26
  constraint equal L12 L26
  constraint vertical L27
  constraint perpendicular L27 L28
  constraint perpendicular L28 L29
  constraint perpendicular L29 L30
  constraint midpoint L27 L31.start
  constraint midpoint L29 L31.end
  constraint midpoint L26.end L31
  constraint equal L24 L28
  measures "d119" distance of L11.end L12.end
  measures "d120" distance of L17.end L18.end
  measures "d121" distance of L19.end L20.end
  measures "d123" distance of L1 L15
  measures "d127" distance of L28.end L29.end
extrude "Extrude13" cut sketch "Sketch14" against normal blind 0.8 contours L13 L14 L15 L16 L17 L18 L19 L20 L21 L22 L23 L24 | L27 L28 L29 L30 bodies 3 in component "Cover"
chamfer "Chamfer1" distance 0.4 angle 45 9 edges at (-0.6887, 30.523, 10.6) (14.048, 31.3343, 10.6) (28.5716, 30.7151, 10.6) (-1.5, 25.0493, 10.6) (29.596, 9.7258, 10.6) (28.7847, -0.6414, 10.6) (14.048, -1.4527, 10.6) (-0.6887, -0.6414, 10.6) (-1.5, 4.2323, 10.6) on bodies 3 in component "Cover"
sketch "Sketch9" plane through (0, 0, 9) normal (0, 0, 1) x (-1, 0, 0) in component "Cover"
  circle A0 centre (-4.5, -3.5473) radius 2.9
  circle A1 centre (-4.5, -3.5473) radius 1.65
  circle A2 centre (-23.596, -14.865) radius 2.9
  circle A3 centre (-23.596, -14.865) radius 1.65
  circle A4 centre (-4.5, -26.5343) radius 1.65
  circle A5 centre (-4.5, -26.5343) radius 2.9
  line L0 (-6.15, -1.1625) -> (-6.15, -5.9321)
  line L1 (-2.85, -1.1625) -> (-2.85, -5.9321)
  line L2 (-25.9808, -13.215) -> (-21.2112, -13.215)
  line L3 (-25.9808, -16.515) -> (-21.2112, -16.515)
  line L4 (-6.15, -24.1495) -> (-6.15, -28.9191)
  line L5 (-2.85, -24.1495) -> (-2.85, -28.9191)
  constraint coincident A0 L0.start
  constraint vertical L0
  constraint coincident A0 L1.end
  constraint coincident A2 L2.start
  constraint coincident A2 L2.end
  constraint parallel L2 L3
  constraint coincident A5 L4.start
  constraint coincident A5 L4.end
  constraint vertical L4
  constraint coincident A5 L5.end
  constraint parallel L4 L5
  constraint tangent A1 L1
  constraint tangent A1 L0
  constraint coincident A0 L0.end
  constraint coincident A2 L3.start
  constraint coincident A5 L5.start
  constraint coincident A2 L3.end
  constraint coincident A0 L1.start
  constraint vertical L1
  constraint tangent A3 L2
  constraint tangent A3 L3
  constraint tangent A4 L4
  constraint tangent A4 L5
  constraint horizontal L2
extrude "Extrude8'" add sketch "Sketch9" along normal blind 0.2 contours A0 L1 | A0 L0 | A2 L2 | A2 L3 | A5 L5 | A5 L4 bodies 3 in component "Cover"
sketch "Sketch10" plane through (0, 0, 9) normal (0, 0, 1) x (-1, 0, 0) in component "Cover"
  line L0 (-23.596, -13.215) -> (-25.9808, -13.215)
  arc A0 (-25.9808, -13.215) -> (-25.9808, -16.515) centre (-23.596, -14.865) ccw
  line L1 (-25.9808, -16.515) -> (-23.596, -16.515)
  arc A1 (-23.596, -13.215) -> (-23.596, -16.515) centre (-23.596, -14.865) ccw
  line L2 (-21.2112, -13.215) -> (-23.596, -13.215)
  arc A2 (-23.596, -16.515) -> (-23.596, -13.215) centre (-23.596, -14.865) ccw
  line L3 (-23.596, -16.515) -> (-21.2112, -16.515)
  arc A3 (-21.2112, -16.515) -> (-21.2112, -13.215) centre (-23.596, -14.865) ccw
  line L4 (-6.15, -1.1625) -> (-6.15, -3.5473)
  arc A4 (-2.85, -3.5473) -> (-6.15, -3.5473) centre (-4.5, -3.5473) ccw
  line L5 (-2.85, -3.5473) -> (-2.85, -1.1625)
  arc A5 (-2.85, -1.1625) -> (-6.15, -1.1625) centre (-4.5, -3.5473) ccw
  line L6 (-6.15, -3.5473) -> (-6.15, -5.9321)
  arc A6 (-6.15, -5.9321) -> (-2.85, -5.9321) centre (-4.5, -3.5473) ccw
  line L7 (-2.85, -5.9321) -> (-2.85, -3.5473)
  arc A7 (-6.15, -3.5473) -> (-2.85, -3.5473) centre (-4.5, -3.5473) ccw
  line L8 (-2.85, -26.5343) -> (-2.85, -24.1495)
  arc A8 (-2.85, -24.1495) -> (-6.15, -24.1495) centre (-4.5, -26.5343) ccw
  line L9 (-6.15, -24.1495) -> (-6.15, -26.5343)
  arc A9 (-2.85, -26.5343) -> (-6.15, -26.5343) centre (-4.5, -26.5343) ccw
  line L10 (-2.85, -28.9191) -> (-2.85, -26.5343)
  arc A10 (-6.15, -26.5343) -> (-2.85, -26.5343) centre (-4.5, -26.5343) ccw
  line L11 (-6.15, -26.5343) -> (-6.15, -28.9191)
  arc A11 (-6.15, -28.9191) -> (-2.85, -28.9191) centre (-4.5, -26.5343) ccw
  line L12 (-25.246, -13.215) -> (-25.246, -16.515)
  line L13 (-21.946, -13.215) -> (-21.946, -16.515)
  line L14 (-6.15, -1.8973) -> (-2.85, -1.8973)
  line L15 (-6.15, -5.1973) -> (-2.85, -5.1973)
  line L16 (-6.15, -24.8843) -> (-2.85, -24.8843)
  line L17 (-6.15, -28.1843) -> (-2.85, -28.1843)
  constraint coincident L0 L12.start
  constraint coincident L1 L12.end
  constraint perpendicular L1 L12
  constraint coincident L2 L13.start
  constraint coincident L3 L13.end
  constraint perpendicular L3 L13
  constraint coincident L4 L14.start
  constraint coincident L5 L14.end
  constraint perpendicular L5 L14
  constraint coincident L6 L15.start
  constraint coincident L7 L15.end
  constraint perpendicular L7 L15
  constraint coincident L9 L16.start
  constraint coincident L8 L16.end
  constraint perpendicular L8 L16
  constraint coincident L11 L17.start
  constraint coincident L10 L17.end
  constraint perpendicular L10 L17
  constraint tangent A10 L17
  constraint tangent A9 L16
  constraint tangent A2 L13
  constraint tangent A1 L12
  constraint tangent A7 L15
  constraint tangent A4 L14
extrude "Extrude9" cut sketch "Sketch10" against normal blind 0.2 contours L0 A1 L12 | L2 A2 L13 | L1 A1 L12 | A2 L3 L13 | L4 A4 L14 | L6 A7 L15 | A4 L5 L14 | L7 A7 L15 | L8 A9 L16 | L10 A10 L17 | L9 A9 L16 | A10 L11 L17 bodies 3 in component "Cover"
chamfer "Chamfer2'" distance 0.4 angle 45 4 edges at (7.2037, 25.4856, 10.6) (7.2037, 2.4986, 10.6) (26.2997, 13.8163, 10.6) (18.796, 23.6343, 10.6) on bodies 3 in component "Cover"
sketch "Sketch11" plane through (0, 0, 2.2) normal (0, 0, -1) x (1, 0, 0) in component "Cover"
  line L0 (28.1942, -0.5473) -> (29.4868, -0.5473)
  arc A0 (29.4868, -0.5473) -> (26.826, 1.4527) centre (26.826, -1.3173) ccw
  line L1 (26.826, 1.4527) -> (1.27, 1.4527)
  arc A1 (1.27, 1.4527) -> (-1.5, -1.3173) centre (1.27, -1.3173) ccw
  line L2 (-1.5, -1.3173) -> (-1.5, -7.1473)
  line L3 (-1.5, -7.1473) -> (-0.3, -7.1473)
  line L4 (-0.3, -7.1473) -> (-0.3, -6.1473)
  line L5 (-0.3, -6.1473) -> (4.5, -6.1473)
  arc A2 (4.5, -6.1473) -> (7.1, -3.5473) centre (4.5, -3.5473) ccw
  line L6 (7.1, -3.5473) -> (7.1, 0.2527)
  line L7 (7.1, 0.2527) -> (26.826, 0.2527)
  arc A3 (28.1942, -0.5473) -> (26.826, 0.2527) centre (26.826, -1.3173) ccw
  circle A4 centre (4.5, -3.5473) radius 1.65
  line L8 (29.5367, -29.1343) -> (28.2889, -29.1343)
  arc A5 (26.826, -30.1343) -> (28.2889, -29.1343) centre (26.826, -28.5643) ccw
  line L9 (26.826, -30.1343) -> (7.1, -30.1343)
  line L10 (7.1, -30.1343) -> (7.1, -26.5343)
  arc A6 (7.1, -26.5343) -> (4.5, -23.9343) centre (4.5, -26.5343) ccw
  line L11 (4.5, -23.9343) -> (-0.3, -23.9343)
  line L12 (-0.3, -23.9343) -> (-0.3, -21.5343)
  line L13 (-0.3, -21.5343) -> (-1.5, -21.5343)
  line L14 (-1.5, -21.5343) -> (-1.5, -28.5643)
  arc A7 (-1.5, -28.5643) -> (1.27, -31.3343) centre (1.27, -28.5643) ccw
  line L15 (1.27, -31.3343) -> (26.826, -31.3343)
  arc A8 (26.826, -31.3343) -> (29.5367, -29.1343) centre (26.826, -28.5643) ccw
  circle A9 centre (4.5, -26.5343) radius 1.65
  line L16 (28.396, -18.1343) -> (29.596, -18.1343)
  line L17 (29.596, -18.1343) -> (29.596, -9.7473)
  line L18 (29.596, -9.7473) -> (28.396, -9.7473)
  line L19 (28.396, -9.7473) -> (28.396, -12.265)
  line L20 (28.396, -12.265) -> (23.596, -12.265)
  arc A10 (23.596, -12.265) -> (23.596, -17.465) centre (23.596, -14.865) ccw
  line L21 (23.596, -17.465) -> (28.396, -17.465)
  line L22 (28.396, -17.465) -> (28.396, -18.1343)
  circle A11 centre (23.596, -14.865) radius 1.65
  line L23 (28.396, -12.265) -> (28.396, -17.465)
  line L24 (7.1, 0.2527) -> (1.7, 0.2527)
  line L25 (-0.3, -23.9343) -> (-0.3, -28.1343)
  line L26 (7.1, -30.1343) -> (1.7, -30.1343)
  line L27 (-0.3, -6.1473) -> (-0.3, -1.7473)
  arc A12 (1.7, 0.2527) -> (-0.3, -1.7473) centre (1.7, -1.7473) ccw
  arc A13 (-0.3, -28.1343) -> (1.7, -30.1343) centre (1.7, -28.1343) ccw
  dimension "d90" = 2
  dimension "d91" = 2
  constraint coincident L19.end L20.start
  constraint coincident L21.end L22.start
  constraint coincident L6.end L7.start
  constraint perpendicular L6 L24
  constraint coincident L11.end L12.start
  constraint perpendicular L11 L25
  constraint coincident L9.end L10.start
  constraint perpendicular L10 L26
  constraint coincident L4.end L5.start
  constraint perpendicular L5 L27
  constraint tangent L24 A12
  constraint tangent L27 A12
  constraint tangent L25 A13
  constraint tangent L26 A13
  measures "d90" radius of A12
  measures "d91" radius of A13
extrude "Extrude10'" add sketch "Sketch11" along normal blind 0.2 contours L0 A0 L1 A1 L2 L3 L4 L7 A3 L24 L27 A12 | L8 A5 L9 L12 L13 L14 A7 L15 A8 L25 L26 A13 | L16 L17 L18 L19 L22 L23 bodies 3 in component "Cover"